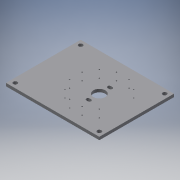
# Autodesk Inventor part: pcb rotary control
Saved by Autodesk Inventor 2016 (Build 200138000, 138)
## iProperties
Created: 2015-10-19
Part Number: pcb rotary control
Material: Generic
Document SubType Name: Sheet Metal
Designer: jeremyhale
Density: 1 g/cm^3
Sheet Metal Rule: Default
Appearance: Default
Author: jeremyhale
Autodesk Inventor part; units mm, degrees
ref_plane "YZ Plane" through (0, 0, 0) normal (1, 0, 0) x (0, 1, 0)
ref_plane "XZ Plane" through (0, 0, 0) normal (0, 1, 0) x (-1, 0, 0)
ref_plane "XY Plane" through (0, 0, 0) normal (0, 0, 1) x (1, 0, 0)
sketch "Sketch1" plane through (0, 0, 0) normal (0, 1, 0) x (-1, 0, 0)
  line L0 (-25, 20) -> (25, 20)
  line L1 (25, 20) -> (25, -20)
  line L2 (25, -20) -> (-25, -20)
  line L3 (-25, -20) -> (-25, 20)
  line L4 (-25, 20) -> (25, -20) construction
  line L5 (25, 20) -> (-25, -20) construction
  point P0 (0, 0)
  dimension "d0" = 50
  dimension "d1" = 40
  constraints: 12 end point, 2 midpoint, 2 parallel, 1 horizontal, 1 perpendicular
  measures "d0" distance of L1.end L2.end
  measures "d1" distance of L0.end L1.end
extrude "Extrusion1" add sketch "Sketch1" along normal blind 1.5875
hole "Hole1" at (22.5, 1.5875, 17.5) direction (0, -1, 0) diameter 2.2 end through all
ref_plane "Work Plane1" through (0, 0, 20) normal (1, 0, 0) x (0, 0, -1)
ref_plane "Work Plane2" through (-25, 0, 0) normal (0, 0, 1) x (1, 0, 0)
mirror "Mirror1" about plane through (0, 0, 20) normal (1, 0, 0) of "Hole1"
mirror "Mirror2" about plane through (-25, 0, 0) normal (0, 0, 1) of "Hole1", "Mirror1"
sketch "Sketch2" plane through (0, 1.5875, 0) normal (0, 1, 0) x (1, 0, 0)
  line L0 (25, -20) -> (25, 20) projected
  line L1 (5, 0) -> (14.1924, -9.1924) construction
  line L2 (5, 0) -> (18, 0) construction
  line L3 (25, 20) -> (-25, 20) construction
  line L4 (5, 0) -> (8.3646, -12.557) construction
  line L5 (5, 0) -> (1.6354, -12.557) construction
  line L6 (5, 0) -> (-4.1924, -9.1924) construction
  line L7 (5, 0) -> (-7.557, -3.3646) construction
  line L8 (5, 0) -> (-7.557, 3.3646) construction
  line L9 (5, 0) -> (-4.1924, 9.1924) construction
  line L10 (5, 0) -> (1.6354, 12.557) construction
  line L11 (5, 0) -> (8.3646, 12.557) construction
  line L12 (5, 0) -> (14.1924, 9.1924) construction
  line L13 (14.1924, -9.1924) -> (12.1604, -7.1604) construction
  circle A0 centre (12.1604, -7.1604) radius 0.305
  circle A1 centre (16.2244, -11.2244) radius 0.305
  circle A2 centre (6.3326, -10.525) radius 0.305
  circle A3 centre (10.3966, -14.589) radius 0.305
  circle A4 centre (-0.3966, -10.525) radius 0.305
  circle A5 centre (3.6674, -14.589) radius 0.305
  circle A6 centre (-6.2244, -7.1604) radius 0.305
  circle A7 centre (-2.1604, -11.2244) radius 0.305
  circle A8 centre (-9.589, -1.3326) radius 0.305
  circle A9 centre (-5.525, -5.3966) radius 0.305
  circle A10 centre (-9.589, 5.3966) radius 0.305
  circle A11 centre (-5.525, 1.3326) radius 0.305
  circle A12 centre (-6.2244, 11.2244) radius 0.305
  circle A13 centre (-2.1604, 7.1604) radius 0.305
  circle A14 centre (-0.3966, 14.589) radius 0.305
  circle A15 centre (3.6674, 10.525) radius 0.305
  circle A16 centre (6.3326, 14.589) radius 0.305
  circle A17 centre (10.3966, 10.525) radius 0.305
  circle A18 centre (12.1604, 11.2244) radius 0.305
  circle A19 centre (16.2244, 7.1604) radius 0.305
  point P0 (0, 0)
  dimension "d14" = 20
  dimension "d15" = 13
  dimension "d16" = 45
  dimension "d17" = 20
  dimension "d20" = 270
  dimension "d22" = 2.032
  dimension "d23" = 2.032
  dimension "d24" = 0.61
  dimension "d27" = 360
  dimension "d33" = 0.61
  dimension "d38" = 0.61
  dimension "d43" = 0.61
  dimension "d48" = 0.61
  dimension "d53" = 0.61
  dimension "d58" = 0.61
  dimension "d63" = 0.61
  dimension "d68" = 0.61
  dimension "d73" = 0.61
  constraints: 24 end point, 20 centre point, 2 coincident, 1 equal length, 1 horizontal, 32 other
  measures "d14" distance from line of L0 L1.start
  measures "d15" distance of L1.start L1.end
  measures "d16" angle of L1 L2
  measures "d17" distance from line of L3 L1.start
  measures "d22" horizontal distance of L13.end L1.end
  measures "d23" horizontal distance of L13.end L1.end
  measures "d24" diameter of A0
  measures "d33" diameter of A2
  measures "d38" diameter of A4
  measures "d43" diameter of A6
  measures "d48" diameter of A8
  measures "d53" diameter of A10
  measures "d58" diameter of A12
  measures "d63" diameter of A14
  measures "d68" diameter of A16
  measures "d73" diameter of A18
hole "Hole2" at (16.2244, 1.5875, 11.2244) at (12.1604, 1.5875, 7.1604) at (16.2244, 1.5875, -7.1604) at (10.3966, 1.5875, 14.589) at (6.3326, 1.5875, 10.525) at (3.6674, 1.5875, 14.589) at (-0.3966, 1.5875, 10.525) at (-2.1604, 1.5875, 11.2244) at (-5.525, 1.5875, 5.3966) at (-6.2244, 1.5875, 7.1604) at (-9.589, 1.5875, 1.3326) at (-5.525, 1.5875, -1.3326) at (-9.589, 1.5875, -5.3966) at (-2.1604, 1.5875, -7.1604) at (-6.2244, 1.5875, -11.2244) at (-0.3966, 1.5875, -14.589) at (3.6674, 1.5875, -10.525) at (6.3326, 1.5875, -14.589) at (10.3966, 1.5875, -10.525) at (12.1604, 1.5875, -11.2244) direction (0, -1, 0) diameter 0.61 end through all
sketch "Sketch3" plane through (0, 1.5875, 0) normal (0, 1, 0) x (1, 0, 0)
  line L0 (25, 20) -> (-25, 20) projected
  line L1 (25, -20) -> (25, 20) projected
  line L2 (5, 0) -> (5, -5.7) construction
  line L3 (5.4, -6.6) -> (4.6, -6.6)
  line L4 (4.6, -6.6) -> (4.6, -4.8)
  line L5 (4.6, -4.8) -> (5.4, -4.8)
  line L6 (5.4, -4.8) -> (5.4, -6.6)
  line L7 (5.4, -6.6) -> (4.6, -4.8) construction
  line L8 (4.6, -6.6) -> (5.4, -4.8) construction
  circle A0 centre (4.6, -5.7) radius 0.9
  circle A1 centre (5.4, -5.7) radius 0.9
  point P0 (0, 0)
  dimension "d81" = 20
  dimension "d82" = 20
  dimension "d83" = 5.7
  dimension "d86" = 0.8
  dimension "d87" = 1.8
  constraints: 14 end point, 4 midpoint, 2 parallel, 2 vertical alignment, 1 horizontal, 1 perpendicular, 1 vertical, 4 other
  measures "d81" distance from line of L0 L2.start
  measures "d82" distance from line of L1 L2.start
  measures "d83" distance of L2.start L2.end
  measures "d86" distance of L4.end L5.end
  measures "d87" distance of L3.end L4.end
extrude "Cut1" cut sketch "Sketch3" against normal blind 3.048
mirror "Mirror3" about plane through (-25, 0, 0) normal (0, 0, 1) of "Cut1"
hole "Hole3" at (5, 1.5875, 0.0102) direction (0, -1, 0) diameter 6.35 depth 3.048 tip angle 118
equation "\"d88\" = Thickness"
equation "\"d97\" = Thickness"
equation "\"BendRadius\" = Thickness"
equation "\"BendReliefWidth\" = Thickness"
equation "\"BendReliefDepth\" = 0.5 * Thickness"
equation "\"CornerReliefSize\" = 4 * Thickness"
equation "\"MinimumRemnant\" = 2 * Thickness"
equation "\"TransitionRadius\" = BendRadius"
equation "\"JacobiRadiusSize\" = Thickness"
equation "\"GapSize\" = Thickness"
equation "\"Thickness\" = 3.048"
body "Solid1"
